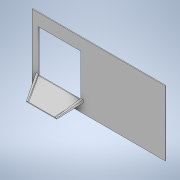
# Autodesk Inventor part: LexanToIntake
Saved by Autodesk Inventor 2020 (Build 240168000, 168)
## iProperties
Created: 2020-01-25
Part Number: LexanToIntake
Material: Generic
Document SubType Name: Modeling
Designer: aidan
Density: 1 g/cm^3
Appearance: Default
Author: aidan
Autodesk Inventor part; units mm, degrees
ref_plane "YZ Plane" through (0, 0, 0) normal (1, 0, 0) x (0, 1, 0)
ref_plane "XZ Plane" through (0, 0, 0) normal (0, 1, 0) x (-1, 0, 0)
ref_plane "XY Plane" through (0, 0, 0) normal (0, 0, 1) x (1, 0, 0)
sketch "Sketch1" plane through (0, 0, 0) normal (0, 0, 1) x (1, 0, 0)
  line L0 (-273.3784, 117.4202) -> (285.4216, 117.4202)
  line L1 (285.4216, 117.4202) -> (285.4216, -155.6298)
  line L2 (285.4216, -155.6298) -> (-273.3784, -155.6298)
  line L3 (-273.3784, -155.6298) -> (-273.3784, 117.4202)
  point P0 (0, 0)
  dimension "d0" = 558.8
  dimension "d1" = 273.05
  constraints: 8 end point, 2 parallel, 1 horizontal, 1 perpendicular
  measures "d0" distance of L0.start L0.end
  measures "d1" distance of L2.end L0.start
extrude "Extrusion1" add sketch "Sketch1" along normal blind 3.175
sketch "Sketch2" plane through (0, 0, 3.175) normal (0, 0, 1) x (1, 0, 0)
  line L0 (-227.9245, -155.6298) -> (-55.3789, -155.6298)
  line L1 (285.4216, 117.4202) -> (-273.3784, 117.4202) projected
  line L2 (-246.8394, 66.6202) -> (-69.0394, 66.6202)
  line L3 (-69.0394, 66.6202) -> (-69.0394, -111.1798)
  line L4 (-69.0394, -111.1798) -> (-246.8394, -111.1798)
  line L5 (-246.8394, -111.1798) -> (-246.8394, 66.6202)
  point P0 (0, 0)
  dimension "d6" = 177.8
  dimension "d7" = 177.8
  dimension "d11" = 50.8
  dimension "d12" = 44.45
  constraints: 10 end point, 2 horizontal, 2 parallel, 1 perpendicular
  measures "d6" distance of L2.start L2.end
  measures "d7" distance of L2.end L3.end
  measures "d11" distance between parallel lines of L1 L2
  measures "d12" distance between parallel lines of L0 L4
extrude "Extrusion2" cut sketch "Sketch2" against normal blind 25.4
ref_plane "Work Plane2" through (0, 0, 79.375) normal (0, 0, 1) x (1, 0, 0)
sketch "Sketch5" plane through (0, 0, 3.175) normal (0, 0, 1) x (1, 0, 0)
  line L0 (-69.0394, -111.1798) -> (-246.8394, -111.1798) projected
  line L1 (-246.8394, -111.1798) -> (-69.0394, -111.1798)
  line L2 (-69.0394, -117.5298) -> (-246.8394, -117.5298)
  line L3 (-246.8394, -117.5298) -> (-256.3644, -117.5298)
  line L4 (-256.3644, -117.5298) -> (-256.3644, -104.8298)
  line L5 (-256.3644, -104.8298) -> (-246.8394, -104.8298)
  line L6 (-246.8394, -111.1798) -> (-246.8394, 66.6202) projected
  line L7 (-69.0394, -117.5298) -> (-59.5144, -117.5298)
  line L8 (-59.5144, -117.5298) -> (-59.5144, -104.8298)
  line L9 (-59.5144, -104.8298) -> (-69.0394, -104.8298)
  line L10 (-69.0394, 66.6202) -> (-69.0394, -111.1798) projected
  line L11 (-69.0394, -111.1798) -> (-69.0394, 66.6202) projected
  line L12 (-246.8394, -117.5298) -> (-69.0394, -117.5298)
  line L13 (-69.0394, -111.1798) -> (-246.8394, -111.1798)
  line L14 (-69.0394, -104.8298) -> (-59.5144, -104.8298)
  line L15 (-59.5144, -104.8298) -> (-59.5144, -117.5298)
  line L16 (-59.5144, -117.5298) -> (-69.0394, -117.5298)
  line L17 (-69.0394, -111.1798) -> (-69.0394, -104.8298)
  line L18 (-256.3644, -104.8298) -> (-246.8394, -104.8298)
  line L19 (-246.8394, -104.8298) -> (-246.8394, -111.1798)
  line L20 (-246.8394, -117.5298) -> (-256.3644, -117.5298)
  line L21 (-256.3644, -117.5298) -> (-256.3644, -104.8298)
  line L22 (-246.8394, -104.8298) -> (-246.8394, -111.1798)
  line L23 (-246.8394, -111.1798) -> (-246.8394, -104.8298)
  point P0 (0, 0)
  dimension "d15" = 9.525
  dimension "d16" = 12.7
  dimension "d18" = 12.7
  dimension "d21" = 6.35
  constraints: 40 end point, 6 horizontal, 6 parallel, 6 perpendicular, 3 point on line, 2 collinear
  measures "d15" distance of L4.end L5.end
  measures "d16" distance of L3.end L4.end
  measures "d18" distance of L7.end L8.end
  measures "d21" distance between parallel lines of L2 L0
sketch "Sketch6" plane through (0, 0, 79.375) normal (0, 0, 1) x (1, 0, 0)
  line L0 (-69.0394, -111.1798) -> (-246.8394, -111.1798) projected
  line L1 (-273.3784, -155.6298) -> (285.4216, -155.6298) projected
  line L2 (-246.8394, -155.6298) -> (-69.0394, -155.6298)
  line L3 (-221.4394, -155.6298) -> (-94.4394, -155.6298)
  line L4 (-94.4394, -155.6298) -> (-94.4394, -152.4548)
  line L5 (-94.4394, -152.4548) -> (-221.4394, -152.4548)
  line L6 (-221.4394, -152.4548) -> (-221.4394, -155.6298)
  point P0 (0, 0)
  dimension "d19" = 25.4
  dimension "d20" = 25.4
  dimension "d26" = 3.175
  constraints: 10 end point, 3 point on line, 2 parallel, 1 horizontal, 1 perpendicular
  measures "d19" distance from line of L6 L0.end
  measures "d20" distance from line of L0.start L4
  measures "d26" distance between parallel lines of L1 L5
loft "Loft1" add profiles "Sketch5", "Sketch6"
equation "\"d0\" = L0"
equation "\"d1\" = W0"
equation "\"L0\" = 558.8"
equation "\"W0\" = 273.05"
body "Solid1"
